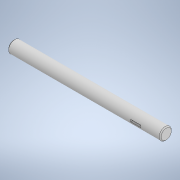
# Autodesk Inventor part: Mainpulo
Saved by Autodesk Inventor 2021 (Build 250183000, 183)
## iProperties
Created: 2022-02-22
Part Number: Mainpulo
Material: Genérico
Document SubType Name: Modeling
Designer: aluno
Density: 1 g/cm^3
Appearance: Padrão
Author: aluno
Autodesk Inventor part; units mm, degrees
ref_plane "YZ Plane" through (0, 0, 0) normal (1, 0, 0) x (0, 1, 0)
ref_plane "XZ Plane" through (0, 0, 0) normal (0, 1, 0) x (-1, 0, 0)
ref_plane "XY Plane" through (0, 0, 0) normal (0, 0, 1) x (1, 0, 0)
sketch "Esboço1" plane through (0, 0, 0) normal (0, 0, 1) x (1, 0, 0)
  line L0 (0, 0) -> (75, 0)
  line L1 (75, 0) -> (75, 3)
  line L2 (75, 3) -> (0, 3)
  line L3 (0, 3) -> (0, 0)
  dimension "d0" = 75
  dimension "d1" = 3
  constraints: 8 end point, 2 parallel, 1 horizontal, 1 perpendicular
  measures "d0" distance of L2.end L1.end
  measures "d1" distance of L1.end L0.end
revolve "Revolução1" add sketch "Esboço1" angle 360 about axis through (0, 0, 0) along (1, 0, 0)
sketch "Esboço2" plane through (0, 0, 0) normal (0, 1, 0) x (-1, 0, 0)
  point P0 (0, 0)
chamfer "Chanfro1" distance 0.5 angle 45 2 edges at (0, -3, 0) (75, -3, 0)
sketch "Esboço3" plane through (0, 0, 0) normal (0, 1, 0) x (-1, 0, 0)
  line L0 (0, 2.5) -> (0, -2.5) projected
  line L1 (-75, 2.5) -> (-74.5, 3) projected
  line L2 (-74.5, 3) -> (-0.5, 3) projected
  line L3 (-0.5, 3) -> (0, 2.5) projected
  line L4 (0, 2.5) -> (0, -2.5) projected
  line L5 (0, -2.5) -> (-0.5, -3) projected
  line L6 (-0.5, -3) -> (-74.5, -3) projected
  line L7 (-74.5, -3) -> (-75, -2.5) projected
  line L8 (-75, -2.5) -> (-75, 2.5) projected
  arc A0 (-9.5, -2) -> (-14.5, -2) centre (-12, -2) ccw
  line L9 (-65.5, 2) -> (-65.5, 3)
  line L10 (-60.5, 3) -> (-60.5, 2)
  arc A1 (-60.7087, 3) -> (-65.2913, 3) centre (-63, 2) ccw
  arc A2 (-65.5, 2) -> (-60.5, 2) centre (-63, 2) ccw
  line L11 (-65.5, 3) -> (-65.2913, 3)
  line L12 (-60.7087, 3) -> (-60.5, 3)
  line L13 (-75, 2.5) -> (-74.5, 3) projected
  line L14 (-74.5, 3) -> (-0.5, 3) projected
  line L15 (-0.5, 3) -> (0, 2.5) projected
  line L16 (0, 2.5) -> (0, -2.5) projected
  line L17 (0, -2.5) -> (-0.5, -3) projected
  line L18 (-0.5, -3) -> (-74.5, -3) projected
  line L19 (-74.5, -3) -> (-75, -2.5) projected
  line L20 (-75, -2.5) -> (-75, 2.5) projected
  line L21 (-0.5, -3) -> (-0.5, 3) projected
  line L22 (-74.5, 3) -> (-74.5, -3) projected
  line L23 (-75, 2.5) -> (-74.5, 3) projected
  line L24 (-74.5, 3) -> (-0.5, 3) projected
  line L25 (-0.5, 3) -> (0, 2.5) projected
  line L26 (0, 2.5) -> (0, -2.5) projected
  line L27 (0, -2.5) -> (-0.5, -3) projected
  line L28 (-0.5, -3) -> (-74.5, -3) projected
  line L29 (-74.5, -3) -> (-75, -2.5) projected
  line L30 (-75, -2.5) -> (-75, 2.5) projected
  line L31 (-14.5, -2) -> (-14.5, -5)
  line L32 (-14.5, -5) -> (-9.5, -5)
  line L33 (-9.5, -5) -> (-9.5, -2)
  point P0 (0, 0)
  point P1 (-14.5, -3)
  point P2 (-9.5, -3)
  point P3 (-14.5, -3)
  point P4 (-9.5, -3)
  dimension "d10" = 12
  dimension "d12" = 12
  dimension "d17" = 2.5
  dimension "d19" = 5
  dimension "d20" = 3
  dimension "d21" = 1
  constraints: 14 end point, 6 point on circle, 3 centre point, 2 perpendicular, 1 parallel, 1 point on line, 1 tangent
  measures "d10" distance from line of L8 A1.centre
  measures "d12" distance from line of L0 A0.centre
  measures "d17" radius of A0
  measures "d19" distance of L32.end L31.end
  measures "d20" distance of L31.end L31.start
  measures "d21" distance from line of A0.centre L18
extrude "Extrusão1" cut sketch "Esboço3" against normal mid plane 1 contours L10 A2 L9 L2 | L6 L31 A0 L33 | L2 A1
